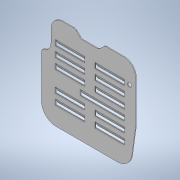
# Autodesk Inventor part: 65. Грязеуловитель
Saved by Autodesk Inventor 2021 (Build 250183000, 183)
## iProperties
Created: 2021-03-10
Part Number: 65. Грязеуловитель
Material: Типовые
Document SubType Name: Modeling
Designer: Данил
Density: 1 g/cm^3
Appearance: По умолчанию
Author: Данил
Autodesk Inventor part; units mm, degrees
ref_plane "YZ Plane" through (0, 0, 0) normal (1, 0, 0) x (0, 1, 0)
ref_plane "XZ Plane" through (0, 0, 0) normal (0, 1, 0) x (-1, 0, 0)
ref_plane "XY Plane" through (0, 0, 0) normal (0, 0, 1) x (1, 0, 0)
sketch "Эскиз1" plane through (0, 0, 0) normal (0, 0, 1) x (1, 0, 0)
  line L0 (-64, 0) -> (64, 0) construction
  line L1 (0, 64) -> (0, -64) construction
  line L2 (-44, -64) -> (39.1656, -64)
  line L3 (-64, -44) -> (-64, 14.1404)
  arc A0 (-64, -44) -> (-44, -64) centre (-44, -44) ccw
  arc A1 (-60.1765, 19) -> (-64, 14.1404) centre (-59, 14.1404) ccw
  arc A2 (-60.1765, 19) -> (-51, 30.6631) centre (-63, 30.6631) ccw
  line L4 (-51, 30.6631) -> (-51, 48)
  line L5 (-35, 64) -> (-20.1421, 64)
  arc A3 (-35, 64) -> (-51, 48) centre (-35, 48) ccw
  line L6 (-16.6066, 62.5355) -> (-11.5355, 57.4645)
  line L7 (-8, 56) -> (12, 56)
  line L8 (15.5355, 57.4645) -> (20.6066, 62.5355)
  line L9 (24.1421, 64) -> (48, 64)
  line L10 (64, 48) -> (64, -11)
  arc A4 (-16.6066, 62.5355) -> (-20.1421, 64) centre (-20.1421, 59) ccw
  arc A5 (-11.5355, 57.4645) -> (-8, 56) centre (-8, 61) ccw
  arc A6 (12, 56) -> (15.5355, 57.4645) centre (12, 61) ccw
  arc A7 (24.1421, 64) -> (20.6066, 62.5355) centre (24.1421, 59) ccw
  arc A8 (64, 48) -> (48, 64) centre (48, 48) ccw
  circle A9 centre (56, 35) radius 2.75
  line L11 (64, -11) -> (58.971, -46.7835)
  arc A10 (39.1656, -64) -> (58.971, -46.7835) centre (39.1656, -44) ccw
  line L12 (9, 38) -> (49, 38)
  line L13 (49, 38) -> (49, 31)
  line L14 (49, 31) -> (9, 31)
  line L15 (9, 31) -> (9, 38)
  line L16 (9, 24) -> (49, 24)
  line L17 (49, 24) -> (49, 17)
  line L18 (49, 17) -> (9, 17)
  line L19 (9, 17) -> (9, 24)
  line L20 (9, 10) -> (49, 10)
  line L21 (49, 10) -> (49, 3)
  line L22 (49, 3) -> (9, 3)
  line L23 (9, 3) -> (9, 10)
  line L24 (-5, 38) -> (-5, 31)
  line L25 (-5, 24) -> (-5, 17)
  line L26 (-45, 38) -> (-5, 38)
  line L27 (-45, 31) -> (-45, 38)
  line L28 (-5, 31) -> (-45, 31)
  line L29 (-45, 24) -> (-5, 24)
  line L30 (-45, 17) -> (-45, 24)
  line L31 (-5, 17) -> (-45, 17)
  line L32 (-45, 10) -> (-5, 10)
  line L33 (-5, 3) -> (-45, 3)
  line L34 (-45, 3) -> (-45, 10)
  line L35 (-5, 10) -> (-5, 3)
  line L36 (-45, -25) -> (-45, -18)
  line L37 (-45, -39) -> (-45, -32)
  line L38 (-5, -25) -> (-45, -25)
  line L39 (-45, -18) -> (-5, -18)
  line L40 (-45, -32) -> (-5, -32)
  line L41 (-5, -39) -> (-45, -39)
  line L42 (-5, -32) -> (-5, -39)
  line L43 (-5, -18) -> (-5, -25)
  line L44 (49, -18) -> (49, -25)
  line L45 (49, -32) -> (49, -39)
  line L46 (9, -39) -> (9, -32)
  line L47 (49, -39) -> (9, -39)
  line L48 (9, -32) -> (49, -32)
  line L49 (49, -25) -> (9, -25)
  line L50 (9, -25) -> (9, -18)
  line L51 (9, -18) -> (49, -18)
  line L52 (-11, -4) -> (49, -4)
  line L53 (49, -4) -> (49, -11)
  line L54 (49, -11) -> (-11, -11)
  line L55 (-11, -11) -> (-11, -4)
  point P0 (0, 0)
  point P1 (0, 0)
  point P2 (-64, -64)
  point P3 (-51, 64)
  point P4 (0, -42)
  dimension "d0" = 128
  dimension "d1" = 20
  dimension "d6" = 13
  dimension "d7" = 5
  dimension "d8" = 12
  dimension "d9" = 45
  dimension "d10" = 16
  dimension "d11" = 5
  dimension "d12" = 45
  dimension "d13" = 45
  dimension "d14" = 20
  dimension "d15" = 8
  dimension "d16" = 16
  dimension "d17" = 52
  dimension "d18" = 5.5
  dimension "d19" = 8
  dimension "d20" = 29
  dimension "d21" = 8
  dimension "d22" = 53
  dimension "d23" = 20
  dimension "d24" = 40
  dimension "d25" = 7
  dimension "d26" = 26
  dimension "d27" = 73
  dimension "d30" = 14
  dimension "d37" = 54
  dimension "d44" = 42
  dimension "d49" = 60
  dimension "d50" = 7
  dimension "d51" = 14
  constraints: 112 end point, 20 point on circle, 19 tangent, 11 centre point, 6 horizontal, 5 parallel, 5 perpendicular, 5 vertical, 4 point on line, 3 equal radius, 3 horizontal alignment, 3 vertical alignment, 2 midpoint, 1 coincident, 73 other
  measures "d0" distance of L0.start L0.end
  measures "d1" radius of A0
  measures "d6" distance between parallel lines of L3 L4
  measures "d7" radius of A1
  measures "d8" radius of A2
  measures "d9" vertical distance of point (-51, 64) A1.start
  measures "d10" radius of A3
  measures "d11" radius of A4
  measures "d12" angle of L7 L8
  measures "d13" angle of L7 L6
  measures "d14" distance of L7.start L7.end
  measures "d15" distance between parallel lines of L9 L7
  measures "d16" radius of A8
  measures "d17" distance from line of L10 L7.end
  measures "d18" diameter of A9
  measures "d19" distance from line of L10 A9.centre
  measures "d20" distance from line of L9 A9.centre
  measures "d21" angle of L10 L11
  measures "d22" distance from line of L2 L10.end
  measures "d23" radius of A10
  measures "d24" distance of L12.start L12.end
  measures "d25" distance of L12.end L13.end
  measures "d26" distance from line of L9 L12.end
  measures "d27" distance from line of L3 L14.end
  measures "d30" distance of L12.start L16.start
  measures "d37" distance of L12.end L24.start
  measures "d44" distance of L29.start L36.end
  measures "d49" distance of L52.start L52.end
  measures "d50" distance of L52.end L53.end
  measures "d51" distance from line of L52 L32.end
extrude "Выдавливание1" add sketch "Эскиз1" along normal mid plane 1
sketch "Эскиз2" plane through (49, 31, 0.5) normal (-1, 0, 0) x (0, 0, 1)
  line L0 (-1, 7) -> (0, 7) projected
  line L1 (0, 7) -> (0, 0) projected
  line L2 (0, 7) -> (-3.3141, 1.2598)
  line L3 (-3.7239, 1.15) -> (-3.9543, 1.283)
  line L4 (-1, 0) -> (-1, 7) projected
  line L5 (-4.0641, 1.6928) -> (-1, 7)
  line L6 (0, -42) -> (0, 17) projected
  arc A0 (-3.7239, 1.15) -> (-3.3141, 1.2598) centre (-3.5739, 1.4098) ccw
  arc A1 (-4.0641, 1.6928) -> (-3.9543, 1.283) centre (-3.8043, 1.5428) ccw
  point P0 (-0.5, -31)
  point P1 (-3.4641, 1)
  dimension "d54" = 30
  dimension "d55" = 6
  dimension "d56" = 0.3
  constraints: 6 end point, 4 point on circle, 4 tangent, 2 centre point, 2 point on line, 1 equal radius, 1 parallel, 1 perpendicular
  measures "d54" angle of L6 L2
  measures "d55" vertical distance of L0.end point (-3.464, 1)
  measures "d56" radius of A0
extrude "Выдавливание2" add sketch "Эскиз2" along normal up to surface (40 mm away)
pattern_linear "Прямоуг.массив1" count 2 spacing 54 along (-1, 0, 0) of "Выдавливание2"
pattern_linear "Прямоуг.массив2" count 3 spacing 14 along (0, -1, 0) of "Выдавливание2", "Прямоуг.массив1"
pattern_linear "Прямоуг.массив3" count 2 spacing 56 along (0, -1, 0) of "Выдавливание2", "Прямоуг.массив1"
pattern_linear "Прямоуг.массив4" count 2 spacing 70 along (0, -1, 0) of "Выдавливание2", "Прямоуг.массив1"
sketch "Эскиз3" plane through (49, -11, 0.5) normal (-1, 0, 0) x (0, 0, 1)
  line L0 (-1, 7) -> (0, 7) projected
  line L1 (0, 7) -> (0, 0) projected
  line L2 (0, 7) -> (-3.3141, 1.2598)
  line L3 (-3.7239, 1.15) -> (-3.9543, 1.283)
  line L4 (-4.0641, 1.6928) -> (-1, 7)
  arc A0 (-3.7239, 1.15) -> (-3.3141, 1.2598) centre (-3.5739, 1.4098) ccw
  arc A1 (-4.0641, 1.6928) -> (-3.9543, 1.283) centre (-3.8043, 1.5428) ccw
  point P0 (-0.5, 11)
  point P1 (-3.4641, 1)
  dimension "d71" = 30
  dimension "d72" = 6
  dimension "d73" = 0.3
  constraints: 6 end point, 4 point on circle, 4 tangent, 2 centre point, 2 point on line, 1 equal radius, 1 parallel, 1 perpendicular
  measures "d71" angle of L1 L2
  measures "d72" vertical distance of L0.end point (-3.464, 1)
  measures "d73" radius of A0
extrude "Выдавливание3" add sketch "Эскиз3" along normal up to surface (60 mm away)
